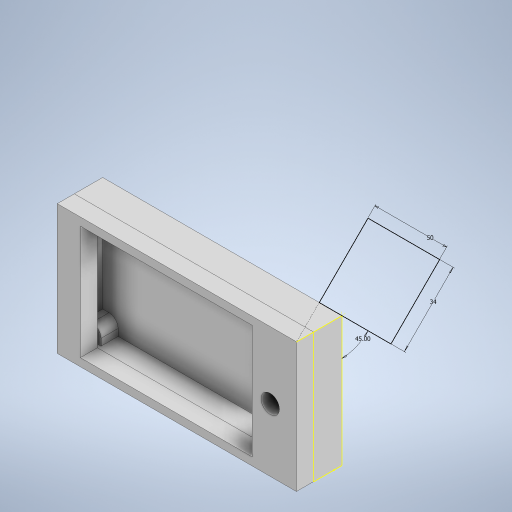
# Autodesk Inventor part: LCD Mount
Saved by Autodesk Inventor 2023.1 (Build 271208000, 208)
## iProperties
Created: 2022-11-09
Part Number: LCD Mount
Material: Generic
Document SubType Name: Modeling
Designer: nicol
Density: 1 g/cm^3
Appearance: Default
Author: nicol
Autodesk Inventor part; units mm, degrees
ref_plane "YZ Plane" through (0, 0, 0) normal (1, 0, 0) x (0, 1, 0)
ref_plane "XZ Plane" through (0, 0, 0) normal (0, 1, 0) x (-1, 0, 0)
ref_plane "XY Plane" through (0, 0, 0) normal (0, 0, 1) x (1, 0, 0)
sketch "Sketch1" plane through (0, 0, 0) normal (0, 0, 1) x (1, 0, 0)
  line L0 (0, 0) -> (118, 0)
  line L1 (118, 0) -> (118, 64)
  line L2 (118, 64) -> (0, 64)
  line L3 (0, 64) -> (0, 0)
  line L4 (4, 60) -> (114, 60)
  line L5 (114, 60) -> (114, 4)
  line L6 (114, 4) -> (4, 4)
  line L7 (4, 4) -> (4, 60)
  dimension "d0" = 110
  dimension "d1" = 56
  dimension "d2" = 4
  constraints: 16 end point, 4 parallel, 2 perpendicular, 1 horizontal, 3 other
  measures "d0" distance of L4.start L4.end
  measures "d1" distance of L6.end L4.start
  measures "d2" distance between parallel lines of L2 L4
extrude "Extrusion1" add sketch "Sketch1" along normal blind 10
extrude "Extrusion2" add sketch "Sketch1" against normal blind 4 contours L3 L2 L1 L0 | L4 L5 L6 L7
sketch "Sketch2" plane through (0, 0, 0) normal (0, 0, 1) x (1, 0, 0)
  line L0 (114, 4) -> (4, 4) projected
  line L1 (4, 4) -> (4, 60) projected
  circle A0 centre (7.1, 56.75) radius 4.4914
  line L2 (114, 60) -> (114, 4) projected
  circle A1 centre (110.9, 56.75) radius 4.4914
  circle A2 centre (110.9, 7.25) radius 4.4914
  circle A3 centre (7.1, 7.25) radius 4.4914
  line L3 (11.5914, 56.75) -> (11.5914, 61.2414)
  line L4 (2.6086, 52.2586) -> (7.1, 52.2586)
  line L5 (106.4086, 60) -> (106.4086, 52.2586)
  line L6 (106.4086, 52.2586) -> (114, 52.2586)
  line L7 (114, 11.7414) -> (106.4086, 11.7414)
  line L8 (106.4086, 11.7414) -> (106.4086, -1.1488)
  line L9 (11.5914, -1.6291) -> (11.5914, 11.7414)
  line L10 (11.5914, 11.7414) -> (2.6086, 11.7414)
  line L11 (4, 4) -> (4, 60) projected
  line L12 (114, 4) -> (4, 4) projected
  line L13 (114, 60) -> (114, 4) projected
  line L14 (4, 60) -> (114, 60) projected
  point P0 (0, 0)
  point P1 (107.8, 60)
  point P2 (106.4086, 56.75)
  point P3 (110.9, 52.2586)
  point P4 (114, 53.5)
  point P5 (106.4086, 7.25)
  point P6 (106.4086, 4)
  point P7 (107.8, 4)
  point P8 (114, 10.5)
  point P9 (110.9, 11.7414)
  point P10 (7.1, 11.7414)
  point P11 (4, 11.7414)
  point P12 (4, 10.5)
  point P13 (10.2, 4)
  point P14 (11.5914, 4)
  point P15 (11.5914, 7.25)
  point P16 (10.2, 60)
  point P17 (4, 53.5)
  point P18 (4, 52.2586)
  point P19 (11.5914, 60)
  dimension "d7" = 103.8
  dimension "d8" = 49.5
  dimension "d9" = 3.25
  dimension "d10" = 3.1
  constraints: 16 end point, 6 vertical, 5 horizontal, 4 coincident, 3 perpendicular, 3 point on circle, 2 horizontal alignment, 2 point on line, 2 tangent, 2 vertical alignment, 1 centre point, 9 other
  measures "d7" distance of point (110.9, 7.25) point (7.1, 7.25)
  measures "d8" distance of point (7.1, 56.75) point (7.1, 7.25)
  measures "d9" distance from line of L0 point (7.1, 7.25)
  measures "d10" distance from line of L1 point (7.1, 7.25)
extrude "Extrusion3" add sketch "Sketch2" along normal blind 8.4 contours A2 L0 | L0 A2 L2 | L2 A2 | L0 L8 A2 | A2 L7 L2 | L0 A3 L9 | L6 A1 L2 | A3 L0 | L0 L1 A3 | A1 L14 L2 | L2 A1 | A3 L1 | A3 L1 L10 | L14 A1 | L5 L14 A1 | L1 A0 L4 | L3 A0 L14 | A0 L1 | L1 L14 A0 | L14 A0
hole "Hole1" at (7.1, 56.75, 0) at (110.9, 56.75, 0) at (110.9, 7.25, 0) at (7.1, 7.25, 0) direction (0, 0, -1) diameter 3.2 end through all both
thicken "Thicken1" operation cut thickness 0.1 both sides no extend neighbours no toward (-1, 0, 0) faces at (4, 25.2471, 5.6) (43.1971, 60, 5.6) (114, 38.7529, 5.6) (74.8029, 4, 2.8)
sketch "Sketch3" plane through (0, 0, 10) normal (0, 0, 1) x (1, 0, 0)
  line L0 (114.1, 60.1) -> (114.1, 3.9) projected
  line L1 (114.1, 3.9) -> (3.9, 3.9) projected
  line L2 (3.9, 3.9) -> (3.9, 60.1) projected
  line L3 (3.9, 60.1) -> (114.1, 60.1) projected
  line L4 (118, 0) -> (118, 64) projected
  line L5 (118, 64) -> (0, 64) projected
  line L6 (0, 64) -> (0, 0) projected
  line L7 (0, 0) -> (118, 0) projected
  line L8 (110.9, 11.7414) -> (114.1, 11.7414) projected
  line L9 (114.1, 52.2586) -> (114.1, 11.7414) projected
  line L10 (114.1, 52.2586) -> (110.9, 52.2586) projected
  arc A0 (106.4086, 56.75) -> (110.9, 52.2586) centre (110.9, 56.75) ccw projected
  line L11 (106.4086, 56.75) -> (106.4086, 60.1) projected
  line L12 (11.5914, 60.1) -> (106.4086, 60.1) projected
  line L13 (11.5914, 60.1) -> (11.5914, 56.75) projected
  arc A1 (7.1, 52.2586) -> (11.5914, 56.75) centre (7.1, 56.75) ccw projected
  line L14 (7.1, 52.2586) -> (3.9, 52.2586) projected
  line L15 (3.9, 11.7414) -> (3.9, 52.2586) projected
  line L16 (3.9, 11.7414) -> (7.1, 11.7414) projected
  arc A2 (11.5914, 7.25) -> (7.1, 11.7414) centre (7.1, 7.25) ccw projected
  line L17 (11.5914, 7.25) -> (11.5914, 3.9) projected
  line L18 (106.4086, 3.9) -> (11.5914, 3.9) projected
  line L19 (106.4086, 3.9) -> (106.4086, 7.25) projected
  arc A3 (110.9, 11.7414) -> (106.4086, 7.25) centre (110.9, 7.25) ccw projected
  line L20 (11.4, 60.1) -> (96.1, 60.1)
  line L21 (96.1, 60.1) -> (96.1, 3.9)
  line L22 (96.1, 3.9) -> (11.4, 3.9)
  line L23 (11.4, 3.9) -> (11.4, 60.1)
  line L24 (114.1, 3.9) -> (3.9, 3.9) projected
  point P0 (96.1, 3.9)
  dimension "d22" = 7.5
  dimension "d23" = 84.7
  constraints: 8 end point, 2 collinear, 2 parallel, 1 horizontal, 1 perpendicular
  measures "d22" distance between parallel lines of L15 L23
  measures "d23" distance of L20.start L20.end
extrude "Extrusion4" add sketch "Sketch3" along normal blind 8.4 separate body contours L0 L10 A0 L11 L3 | L0 L8 A3 L19 L1 L21 L3 L11 A0 L10 | L0 L1 L19 A3 L8 | L23 A1 L14 L2 L3 | L23 A2 L16 L2 L14 A1 | L1 L2 L16 A2 L23 | L7 L6 L5 L4
sketch "Sketch4" plane through (0, 0, 18.4) normal (0, 0, 1) x (1, 0, 0)
  circle A0 centre (105.1, 31) radius 4.5
  line L0 (96.1, 60.1) -> (96.1, 3.9) projected
  point P0 (0, 0)
  point P1 (96.1, 32)
  point P2 (96.1, 32)
  dimension "d26" = 9
  dimension "d27" = 9
  dimension "d30" = 1
  constraints: 2 midpoint, 1 centre point
  measures "d26" distance from line of L0 A0.centre
  measures "d27" diameter of A0
  measures "d30" vertical distance of A0.centre point (96.1, 32)
extrude "Extrusion5" cut sketch "Sketch4" against normal blind 8.4 bodies 2
sketch "Sketch5" plane through (118, 0, 10) normal (1, 0, 0) x (0, 0, -1)
  line L0 (26.8416, 99.2416) -> (62.197, 63.8863)
  line L1 (62.197, 63.8863) -> (38.1553, 39.8447)
  line L2 (38.1553, 39.8447) -> (2.8, 75.2)
  line L3 (2.8, 75.2) -> (26.8416, 99.2416)
  line L4 (0, 64) -> (-8.4, 64) projected
  line L5 (-8.4, 64) -> (26.8416, 99.2416) construction
  line L6 (14, 64) -> (14, 0) projected
  line L7 (14, 64) -> (0, 64) projected
  line L8 (0, 0) -> (0, 64) projected
  line L9 (0, 0) -> (14, 0) projected
  line L10 (14, 64) -> (14, 0) projected
  point P0 (10, 0)
  dimension "d31" = 34
  dimension "d32" = 50
  dimension "d33" = 45
  constraints: 10 end point, 2 parallel, 1 collinear, 1 perpendicular, 1 point on line
  measures "d31" distance of L0.end L1.end
  measures "d32" distance of L0.start L0.end
  measures "d33" angle of L2 L6
body "Solid1"
body "Solid2"
